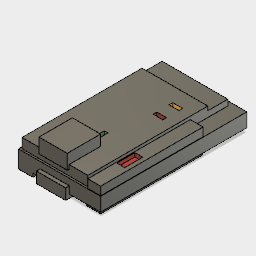
Xdrip PCB (Autodesk Fusion 360 design; units mm, degrees)
Autodesk Fusion 360 part; units mm, degrees
sketch "Sketch1" plane through (0, 0, 0) normal (0, 1, 0) x (1, 0, 0)
  line L0 (0, 0) -> (-22.5, 0)
  line L1 (-22.5, 0) -> (-22.5, -40)
  line L2 (-22.5, -40) -> (0, -40)
  line L3 (0, -40) -> (0, 0)
  dimension "d1" = 40
  dimension "d2" = 22.5
  constraint horizontal L0
  constraint vertical L1
  constraint horizontal L2
  constraint vertical L3
extrude "Extrude1" add sketch "Sketch1" along normal blind 1.8 makes body 1
sketch "Sketch2" plane through (0, 1.8, 0) normal (0, 1, 0) x (-1, 0, 0)
  line L0 (0, 40) -> (0, 0)
  line L1 (0, 0) -> (22.5, 0)
  line L2 (22.5, 0) -> (22.5, 40)
  line L3 (22.5, 40) -> (0, 40)
  line L4 (22, 39.5) -> (4, 39.5)
  line L5 (4, 39.5) -> (4, 1.2)
  line L6 (4, 1.2) -> (22, 1.2)
  line L7 (22, 1.2) -> (22, 39.5)
  dimension "d5" = 18
  dimension "d6" = 38.3
  dimension "d7" = 0.5
  dimension "d8" = 0.5
  constraint horizontal L4
  constraint vertical L5
  constraint horizontal L6
  constraint vertical L7
  measures "d7" distance of L3
  measures "d8" distance of L2
extrude "Extrude2" add sketch "Sketch2" along normal blind 1.6 contours L4 L5 L6 L7 bodies 1
sketch "Sketch3" plane through (0, 3.4, 0) normal (0, 1, 0) x (-1, 0, 0)
  line L0 (22, 1.2) -> (22, 39.5)
  line L1 (22, 39.5) -> (4, 39.5)
  line L2 (4, 39.5) -> (4, 1.2)
  line L3 (4, 1.2) -> (22, 1.2)
  line L4 (16.85, 40.1) -> (9.13, 40.1)
  line L5 (9.13, 40.1) -> (9.13, 30.88)
  line L6 (9.13, 30.88) -> (16.85, 30.88)
  line L7 (16.85, 30.88) -> (16.85, 40.1)
  line L8 (22.5, 40) -> (0, 40)
  constraint horizontal L4
  constraint vertical L5
  constraint horizontal L6
  constraint vertical L7
extrude "Extrude3" add sketch "Sketch3" along normal blind 4 contours L1 L5 L6 L7 bodies 1
extrude "Extrude4" add sketch "Sketch3" along normal blind 4 contours L1 L5 L7 L8 bodies 1
sketch "Sketch4" plane through (0, 3.4, 0) normal (0, 1, 0) x (-1, 0, 0)
  line L0 (9.13, 30.88) -> (9.13, 39.5)
  line L1 (9.13, 39.5) -> (4, 39.5)
  line L2 (4, 39.5) -> (4, 1.2)
  line L3 (4, 1.2) -> (22, 1.2)
  line L4 (22, 1.2) -> (22, 39.5)
  line L5 (22, 39.5) -> (16.85, 39.5)
  line L6 (16.85, 39.5) -> (16.85, 30.88)
  line L7 (16.85, 30.88) -> (9.13, 30.88)
  line L8 (22, 30.7) -> (4, 30.7)
  line L9 (4, 30.7) -> (4, 6.7)
  line L10 (4, 6.7) -> (22, 6.7)
  line L11 (22, 6.7) -> (22, 30.7)
  line L12 (22, 39.5) -> (22, 1.2)
  dimension "d20" = 18
  dimension "d21" = 24
  dimension "d22" = 5.5
  constraint horizontal L8
  constraint vertical L9
  constraint horizontal L10
  constraint vertical L11
  constraint coincident L4
  measures "d22" distance of L3 L10
extrude "Extrude11" add sketch "Sketch4" along normal blind 1.1 contours L2 L4 L8 L9 L10 L11 L12 bodies 1
sketch "Sketch5" plane through (0, 1.8, 0) normal (0, 1, 0) x (-1, 0, 0)
  line L0 (22, 1.2) -> (4, 1.2)
  line L1 (4, 1.2) -> (4, 39.5)
  line L2 (4, 39.5) -> (22, 39.5)
  line L3 (22, 39.5) -> (22, 1.2)
  line L4 (0, 40) -> (0, 0)
  line L5 (0, 0) -> (22.5, 0)
  line L6 (22.5, 0) -> (22.5, 40)
  line L7 (22.5, 40) -> (0, 40)
  line L8 (0.1, 39.9) -> (3.6, 39.9)
  line L9 (3.6, 39.9) -> (3.6, 11.9)
  line L10 (3.6, 11.9) -> (0.1, 11.9)
  line L11 (0.1, 11.9) -> (0.1, 39.9)
  dimension "d25" = 28
  dimension "d26" = 3.5
  dimension "d27" = 0.1
  dimension "d28" = 0.1
  constraint horizontal L8
  constraint vertical L9
  constraint horizontal L10
  constraint vertical L11
  constraint midpoint L8
  measures "d27" distance of L4 L11
  measures "d28" distance of L7
extrude "Extrude6" add sketch "Sketch5" along normal blind 2.3 contours L8 L9 L10 L11 bodies 1
sketch "Sketch6" plane through (0, 0, 0) normal (0, -1, 0) x (1, 0, 0)
  line L0 (0, 0) -> (0, 40)
  line L1 (0, 40) -> (-22.5, 40)
  line L2 (-22.5, 40) -> (-22.5, 0)
  line L3 (-22.5, 0) -> (0, 0)
  line L4 (-8.55, 39.9) -> (-16.55, 39.9)
  line L5 (-16.55, 39.9) -> (-16.55, 34.25)
  line L6 (-16.55, 34.25) -> (-8.55, 34.25)
  line L7 (-8.55, 34.25) -> (-8.55, 39.9)
  dimension "d31" = 8
  dimension "d32" = 5.65
  dimension "d33" = 8.55
  dimension "d34" = 0.1
  constraint horizontal L4
  constraint vertical L5
  constraint horizontal L6
  constraint vertical L7
  constraint midpoint L4
  measures "d33" distance of L0
  measures "d34" distance of L1
extrude "Extrude7" add sketch "Sketch6" along normal blind 3 contours L4 L5 L6 L7 bodies 1
move_face "OffsetFaces1" offset 1.1 1 faces at (-11.2167, -1, 39.9) on bodies 1
move_face "OffsetFaces2" offset -1.1 1 faces at (-13.8833, -1, 34.25) on bodies 1
sketch "Sketch7" plane through (0, 0, 0) normal (0, -1, 0) x (1, 0, 0)
  line L0 (0, 40) -> (-8.55, 40)
  line L1 (-8.55, 40) -> (-8.55, 35.35)
  line L2 (-8.55, 35.35) -> (-16.55, 35.35)
  line L3 (-16.55, 35.35) -> (-16.55, 40)
  line L4 (-16.55, 40) -> (-22.5, 40)
  line L5 (-22.5, 40) -> (-22.5, 0)
  line L6 (-22.5, 0) -> (0, 0)
  line L7 (0, 0) -> (0, 40)
  line L8 (-9.1, 8.8) -> (-1.5, 8.8)
  line L9 (-1.5, 8.8) -> (-1.5, 0.8)
  line L10 (-1.5, 0.8) -> (-9.1, 0.8)
  line L11 (-9.1, 0.8) -> (-9.1, 8.8)
  dimension "d39" = 7.6
  dimension "d40" = 8
  dimension "d41" = 0.8
  dimension "d42" = 1.5
  constraint horizontal L8
  constraint vertical L9
  constraint horizontal L10
  constraint vertical L11
  measures "d41" distance of L6 L10
  measures "d42" distance of L7 L9
extrude "Extrude8" add sketch "Sketch7" along normal blind 2 contours L8 L9 L10 L11 bodies 1
sketch "Sketch8" plane through (0, 0, 0) normal (0, -1, 0) x (1, 0, 0)
  line L0 (-9.1, 0.8) -> (-9.1, 8.8)
  line L1 (-9.1, 8.8) -> (-1.5, 8.8)
  line L2 (-1.5, 8.8) -> (-1.5, 0.8)
  line L3 (-1.5, 0.8) -> (-9.1, 0.8)
  line L4 (0, 40) -> (-8.55, 40)
  line L5 (-8.55, 40) -> (-8.55, 35.35)
  line L6 (-8.55, 35.35) -> (-16.55, 35.35)
  line L7 (-16.55, 35.35) -> (-16.55, 40)
  line L8 (-16.55, 40) -> (-22.5, 40)
  line L9 (-22.5, 40) -> (-22.5, 0)
  line L10 (-22.5, 0) -> (0, 0)
  line L11 (0, 0) -> (0, 40)
  line L12 (-24.05, 5.85) -> (-22.5, 5.85)
  line L13 (-22.5, 5.85) -> (-22.5, 3.05)
  line L14 (-22.5, 3.05) -> (-24.05, 3.05)
  line L15 (-24.05, 3.05) -> (-24.05, 5.85)
  dimension "d45" = 1.55
  dimension "d46" = 2.8
  dimension "d61" = 3.05
  dimension "d62" = 22.5
  constraint horizontal L12
  constraint vertical L13
  constraint horizontal L14
  constraint vertical L15
  measures "d61" distance of L10
  measures "d62" distance of L11
extrude "Extrude9" add sketch "Sketch8" along normal blind 1.1 separate body contours L9 L12 L13 L14 L15 makes body 2
sketch "Sketch9" plane through (0, 0, 0) normal (0, -1, 0) x (1, 0, 0)
  line L0 (-9.1, 0.8) -> (-9.1, 8.8)
  line L1 (-9.1, 8.8) -> (-1.5, 8.8)
  line L2 (-1.5, 8.8) -> (-1.5, 0.8)
  line L3 (-1.5, 0.8) -> (-9.1, 0.8)
  line L4 (0, 40) -> (-8.55, 40)
  line L5 (-8.55, 40) -> (-8.55, 35.35)
  line L6 (-8.55, 35.35) -> (-16.55, 35.35)
  line L7 (-16.55, 35.35) -> (-16.55, 40)
  line L8 (-16.55, 40) -> (-22.5, 40)
  line L9 (-22.5, 40) -> (-22.5, 0)
  line L10 (-22.5, 0) -> (0, 0)
  line L11 (0, 0) -> (0, 40)
  line L12 (-4.1, 11.9) -> (-0.1, 11.9)
  line L13 (-0.1, 11.9) -> (-0.1, 39.9)
  line L14 (-0.1, 39.9) -> (-4.1, 39.9)
  line L15 (-4.1, 39.9) -> (-4.1, 11.9)
  dimension "d51" = 28
  dimension "d52" = 4
  dimension "d63" = 0.1
  dimension "d64" = 0.1
  constraint horizontal L12
  constraint vertical L13
  constraint horizontal L14
  constraint vertical L15
  measures "d63" distance of L11 L13
  measures "d64" distance of L4 L14
extrude "Extrude10" add sketch "Sketch9" along normal blind 2.5 contours L12 L13 L14 L15 bodies 1
move_face "OffsetFaces3" offset 2 1 faces at (-16.05, 0, 14.7167) on bodies 1
move_face "OffsetFaces4" offset 8.8 1 faces at (-10, 4.1333, 30.7) on bodies 1
combine "Combine1" operation add target body 1 tool bodies 2
sketch "Sketch10" plane through (0, -2, 0) normal (0, -1, 0) x (1, 0, 0)
  line L0 (-4.1, 39.9) -> (-0.1, 39.9)
  line L1 (-0.1, 39.9) -> (-0.1, 11.9)
  line L2 (-0.1, 11.9) -> (-4.1, 11.9)
  line L3 (-4.1, 11.9) -> (-4.1, 39.9)
  line L4 (0, 40) -> (-8.55, 40)
  line L5 (-8.55, 40) -> (-8.55, 35.35)
  line L6 (-8.55, 35.35) -> (-16.55, 35.35)
  line L7 (-16.55, 35.35) -> (-16.55, 40)
  line L8 (-16.55, 40) -> (-22.5, 40)
  line L9 (-22.5, 40) -> (-22.5, 0)
  line L10 (-22.5, 0) -> (0, 0)
  line L11 (0, 0) -> (0, 40)
  line L12 (-22.5, 40) -> (-18.5, 40)
  line L13 (-18.5, 40) -> (-18.5, 36)
  line L14 (-18.5, 36) -> (-22.5, 36)
  line L15 (-22.5, 36) -> (-22.5, 40)
  dimension "d65" = 4
  dimension "d66" = 4
  constraint horizontal L12
  constraint vertical L13
  constraint horizontal L14
  constraint vertical L15
extrude "Extrude12" add sketch "Sketch10" along normal blind 1 contours L8 L9 L12 L13 L14 L15 bodies 1
ref_plane "WorkPlane1" through (-11.25, 4.1, 20) normal (0, 1, 0) x (0, 0, 1)
sketch "Sketch11" plane through (0, 1.8, 0) normal (0, 1, 0) x (-1, 0, 0)
  line L0 (0.1, 11.9) -> (0.1, 39.9)
  line L1 (0.1, 39.9) -> (3.6, 39.9)
  line L2 (3.6, 39.9) -> (3.6, 11.9)
  line L3 (3.6, 11.9) -> (0.1, 11.9)
  line L4 (22, 1.2) -> (4, 1.2)
  line L5 (4, 1.2) -> (4, 39.5)
  line L6 (4, 39.5) -> (22, 39.5)
  line L7 (22, 39.5) -> (22, 1.2)
  line L8 (0, 40) -> (0, 0)
  line L9 (0, 0) -> (22.5, 0)
  line L10 (22.5, 0) -> (22.5, 40)
  line L11 (22.5, 40) -> (0, 40)
  line L12 (0, 0) -> (2, 0)
  line L13 (2, 0) -> (2, 2)
  line L14 (2, 2) -> (0, 2)
  line L15 (0, 2) -> (0, 0)
  constraint horizontal L12
  constraint vertical L13
  constraint horizontal L14
  constraint vertical L15
extrude "Extrude13" add sketch "Sketch11" along normal blind 2.3 contours L8 L9 L12 L13 L14 L15 bodies 1
sketch "Sketch12" plane through (-11.25, 4.1, 20) normal (0, 1, 0) x (1, 0, 0)
  line L0 (11.25, 20) -> (10.05, 20)
  line L1 (10.05, 20) -> (10.05, -7.3)
  line L2 (10.05, -7.3) -> (11.25, -7.3)
  line L3 (11.25, -7.3) -> (11.25, 20)
  line L4 (10.05, -7.3) -> (7.9, -7.3)
  line L5 (7.9, -7.3) -> (7.9, -12.2)
  line L6 (7.9, -12.2) -> (10.05, -12.2)
  line L7 (10.05, -12.2) -> (10.05, -7.3)
  dimension "d72" = 27.3
  dimension "d73" = 1.2
  dimension "d74" = 2.15
  dimension "d75" = 4.9
  constraint horizontal L0
  constraint vertical L1
  constraint horizontal L2
  constraint vertical L3
  constraint horizontal L4
  constraint vertical L5
  constraint horizontal L6
  constraint vertical L7
extrude "Extrude14" cut sketch "Sketch12" against normal blind 1 contours L4 L5 L6 L7 bodies 1
move_face "OffsetFaces5" offset 0.4 1 faces at (-0.6667, 4.1, 1.3333) on bodies 1
ref_plane "WorkPlane2" through (-13, 4.5, 23.1) normal (0, 1, 0) x (0, 0, 1)
sketch "Sketch13" plane through (-13, 4.5, 23.1) normal (0, 1, 0) x (1, 0, 0)
  line L0 (13, 23.1) -> (-13, 23.1)
  line L1 (-13, 23.1) -> (-13, 12.4)
  line L2 (-13, 12.4) -> (13, 12.4)
  line L3 (13, 12.4) -> (13, 23.1)
  line L4 (13, 23.1) -> (-13, 23.1)
  line L5 (-13, 23.1) -> (-13, 8)
  line L6 (-13, 8) -> (13, 8)
  line L7 (13, 8) -> (13, 23.1)
  line L8 (13, 23.1) -> (-13, 23.1)
  line L9 (-13, 23.1) -> (-13, -3.6)
  line L10 (-13, -3.6) -> (13, -3.6)
  line L11 (13, -3.6) -> (13, 23.1)
  line L12 (13, 23.1) -> (6.1, 23.1)
  line L13 (6.1, 23.1) -> (6.1, -3.6)
  line L14 (6.1, -3.6) -> (13, -3.6)
  line L15 (13, -3.6) -> (13, 23.1)
  line L16 (13, 23.1) -> (1.7, 23.1)
  line L17 (1.7, 23.1) -> (1.7, -3.6)
  line L18 (1.7, -3.6) -> (13, -3.6)
  line L19 (13, -3.6) -> (13, 23.1)
  line L20 (6.1, 12.4) -> (3.4, 12.4)
  line L21 (3.4, 12.4) -> (3.4, 11.4)
  line L22 (3.4, 11.4) -> (6.1, 11.4)
  line L23 (6.1, 11.4) -> (6.1, 12.4)
  line L24 (6.1, 8) -> (3.4, 8)
  line L25 (3.4, 8) -> (3.4, 7)
  line L26 (3.4, 7) -> (6.1, 7)
  line L27 (6.1, 7) -> (6.1, 8)
  line L28 (1.7, -3.6) -> (0.7, -3.6)
  line L29 (0.7, -3.6) -> (0.7, -6.3)
  line L30 (0.7, -6.3) -> (1.7, -6.3)
  line L31 (1.7, -6.3) -> (1.7, -3.6)
  dimension "d80" = 26
  dimension "d81" = 10.7
  dimension "d82" = 15.1
  dimension "d83" = 26
  dimension "d84" = 26.7
  dimension "d85" = 6.9
  dimension "d86" = 11.3
  dimension "d87" = 1
  dimension "d88" = 2.7
  dimension "d89" = 1
  dimension "d90" = 2.7
  dimension "d91" = 1
  dimension "d92" = 2.7
  constraint horizontal L0
  constraint vertical L1
  constraint horizontal L2
  constraint vertical L3
  constraint horizontal L4
  constraint vertical L5
  constraint horizontal L6
  constraint vertical L7
  constraint vertical L9
  constraint horizontal L10
  constraint vertical L11
  constraint horizontal L12
  constraint vertical L13
  constraint horizontal L14
  constraint horizontal L16
  constraint vertical L17
  constraint horizontal L18
  constraint horizontal L20
  constraint vertical L21
  constraint horizontal L22
  constraint vertical L23
  constraint coincident L13
  constraint coincident L2
  constraint horizontal L24
  constraint vertical L25
  constraint horizontal L26
  constraint vertical L27
  constraint coincident L6
  constraint horizontal L28
  constraint vertical L29
  constraint horizontal L30
  constraint vertical L31
extrude "Extrude15" cut sketch "Sketch13" against normal blind 1 contours L10 L28 L29 L30 L31 bodies 1
extrude "Extrude16" cut sketch "Sketch13" against normal blind 1 contours L6 L13 L24 L25 L26 L27 bodies 1
extrude "Extrude17" cut sketch "Sketch13" against normal blind 1 contours L2 L13 L20 L21 L22 L23 bodies 1
move_face "OffsetFaces6" offset -2.7 1 faces at (-0.6667, 4.5, 1.3333) on bodies 1
